Autodesk Fusion 360 part; units mm, degrees
(part 2 of 2)
sketch "Sketch7" plane through (0, 0, 4) normal (0, 0, 1) x (-1, 0, 0)
  line L0 (44.4952, -43.9167) -> (47.9684, -47.5134)
  arc A0 (45.8104, -49.5974) -> (47.9684, -47.5134) centre (46.8894, -48.5554) ccw
  line L1 (45.8104, -49.5974) -> (42.3371, -46.0007)
  arc A1 (44.4952, -43.9167) -> (42.3371, -46.0007) centre (43.4161, -44.9587) ccw
  line L2 (54.8766, -29.951) -> (59.2067, -32.451)
  arc A2 (57.7067, -35.049) -> (59.2067, -32.451) centre (58.4567, -33.75) ccw
  line L3 (57.7067, -35.049) -> (53.3766, -32.549)
  arc A3 (54.8766, -29.951) -> (53.3766, -32.549) centre (54.1266, -31.25) ccw
  line L4 (56.8322, -26.05) -> (61.3262, -28.2419)
  arc A4 (60.011, -30.9382) -> (61.3262, -28.2419) centre (60.6686, -29.5901) ccw
  line L5 (60.011, -30.9382) -> (55.5171, -28.7464)
  arc A5 (56.8322, -26.05) -> (55.5171, -28.7464) centre (56.1746, -27.3982) ccw
  line L6 (61.811, -9.3758) -> (66.735, -10.244)
  arc A6 (66.2141, -13.1985) -> (66.735, -10.244) centre (66.4745, -11.7213) ccw
  line L7 (66.2141, -13.1985) -> (61.29, -12.3302)
  arc A7 (61.811, -9.3758) -> (61.29, -12.3302) centre (61.5505, -10.853) ccw
  line L8 (58.9775, 20.7401) -> (63.7328, 22.2852)
  arc A8 (64.6598, 19.4321) -> (63.7328, 22.2852) centre (64.1963, 20.8586) ccw
  line L9 (64.6598, 19.4321) -> (59.9046, 17.887)
  arc A9 (58.9775, 20.7401) -> (59.9046, 17.887) centre (59.441, 19.3136) ccw
  circle A10 centre (0, 0) radius 15
  line L10 (60.2806, 16.5756) -> (65.1321, 17.7852)
  arc A11 (65.8578, 14.8743) -> (65.1321, 17.7852) centre (65.495, 16.3297) ccw
  line L11 (65.8578, 14.8743) -> (61.0064, 13.6647)
  arc A12 (60.2806, 16.5756) -> (61.0064, 13.6647) centre (60.6435, 15.1201) ccw
  line L12 (62.0008, 8.0248) -> (66.9734, 8.5475)
  arc A13 (67.287, 5.5639) -> (66.9734, 8.5475) centre (67.1302, 7.0557) ccw
  line L13 (67.287, 5.5639) -> (62.3144, 5.0412)
  arc A14 (62.0008, 8.0248) -> (62.3144, 5.0412) centre (62.1576, 6.533) ccw
  line L14 (61.0064, -13.6647) -> (65.8578, -14.8743)
  arc A15 (65.1321, -17.7852) -> (65.8578, -14.8743) centre (65.495, -16.3297) ccw
  line L15 (65.1321, -17.7852) -> (60.2806, -16.5756)
  arc A16 (61.0064, -13.6647) -> (60.2806, -16.5756) centre (60.6435, -15.1201) ccw
  line L16 (58.5109, -22.0221) -> (63.1468, -23.8952)
  arc A17 (62.023, -26.6767) -> (63.1468, -23.8952) centre (62.5849, -25.2859) ccw
  line L17 (62.023, -26.6767) -> (57.3871, -24.8037)
  arc A18 (58.5109, -22.0221) -> (57.3871, -24.8037) centre (57.949, -23.4129) ccw
  line L18 (57.3871, 24.8037) -> (62.023, 26.6767)
  arc A19 (63.1468, 23.8952) -> (62.023, 26.6767) centre (62.5849, 25.2859) ccw
  line L19 (63.1468, 23.8952) -> (58.5109, 22.0221)
  arc A20 (57.3871, 24.8037) -> (58.5109, 22.0221) centre (57.949, 23.4129) ccw
  line L20 (52.6536, -33.706) -> (56.7988, -36.502)
  arc A21 (55.1212, -38.9891) -> (56.7988, -36.502) centre (55.96, -37.7455) ccw
  line L21 (55.1212, -38.9891) -> (50.9761, -36.1931)
  arc A22 (52.6536, -33.706) -> (50.9761, -36.1931) centre (51.8148, -34.9496) ccw
  line L22 (47.4502, -40.7059) -> (51.166, -44.0516)
  arc A23 (49.1586, -46.281) -> (51.166, -44.0516) centre (50.1623, -45.1663) ccw
  line L23 (49.1586, -46.281) -> (45.4429, -42.9354)
  arc A24 (47.4502, -40.7059) -> (45.4429, -42.9354) centre (46.4466, -41.8207) ccw
  line L24 (62.4096, 3.6803) -> (67.4065, 3.8548)
  arc A25 (67.5112, 0.8566) -> (67.4065, 3.8548) centre (67.4589, 2.3557) ccw
  line L25 (67.5112, 0.8566) -> (62.5143, 0.6821)
  arc A26 (62.4096, 3.6803) -> (62.5143, 0.6821) centre (62.4619, 2.1812) ccw
  line L26 (62.5143, -0.6821) -> (67.5112, -0.8566)
  arc A27 (67.4065, -3.8548) -> (67.5112, -0.8566) centre (67.4589, -2.3557) ccw
  line L27 (67.4065, -3.8548) -> (62.4096, -3.6803)
  arc A28 (62.5143, -0.6821) -> (62.4096, -3.6803) centre (62.4619, -2.1812) ccw
  line L28 (62.3144, -5.0412) -> (67.287, -5.5639)
  arc A29 (66.9734, -8.5475) -> (67.287, -5.5639) centre (67.1302, -7.0557) ccw
  line L29 (66.9734, -8.5475) -> (62.0008, -8.0248)
  arc A30 (62.3144, -5.0412) -> (62.0008, -8.0248) centre (62.1576, -6.533) ccw
  line L30 (55.5171, 28.7464) -> (60.011, 30.9382)
  arc A31 (61.3262, 28.2419) -> (60.011, 30.9382) centre (60.6686, 29.5901) ccw
  line L31 (61.3262, 28.2419) -> (56.8322, 26.05)
  arc A32 (55.5171, 28.7464) -> (56.8322, 26.05) centre (56.1746, 27.3982) ccw
  line L32 (61.29, 12.3302) -> (66.2141, 13.1985)
  arc A33 (66.735, 10.244) -> (66.2141, 13.1985) centre (66.4745, 11.7213) ccw
  line L33 (66.735, 10.244) -> (61.811, 9.3758)
  arc A34 (61.29, 12.3302) -> (61.811, 9.3758) centre (61.5505, 10.853) ccw
  line L34 (59.9046, -17.887) -> (64.6598, -19.4321)
  arc A35 (63.7328, -22.2852) -> (64.6598, -19.4321) centre (64.1963, -20.8586) ccw
  line L35 (63.7328, -22.2852) -> (58.9775, -20.7401)
  arc A36 (59.9046, -17.887) -> (58.9775, -20.7401) centre (59.441, -19.3136) ccw
  circle A37 centre (47.4149, 27.375) radius 2.45
  circle A38 centre (0, -54.75) radius 2.45
  line L36 (53.3766, 32.549) -> (57.7067, 35.049)
  arc A39 (59.2067, 32.451) -> (57.7067, 35.049) centre (58.4567, 33.75) ccw
  line L37 (59.2067, 32.451) -> (54.8766, 29.951)
  arc A40 (53.3766, 32.549) -> (54.8766, 29.951) centre (54.1266, 31.25) ccw
  circle A41 centre (-47.4149, 27.375) radius 2.45
  line L38 (50.9761, 36.1931) -> (55.1212, 38.9891)
  arc A42 (56.7988, 36.502) -> (55.1212, 38.9891) centre (55.96, 37.7455) ccw
  line L39 (56.7988, 36.502) -> (52.6536, 33.706)
  arc A43 (50.9761, 36.1931) -> (52.6536, 33.706) centre (51.8148, 34.9496) ccw
  line L40 (48.3272, 39.6609) -> (52.2672, 42.7392)
  arc A44 (54.1142, 40.3751) -> (52.2672, 42.7392) centre (53.1907, 41.5571) ccw
  line L41 (54.1142, 40.3751) -> (50.1742, 37.2968)
  arc A45 (48.3272, 39.6609) -> (50.1742, 37.2968) centre (49.2507, 38.4788) ccw
  line L42 (24.5122, 4.9145) -> (55.4976, 22.8039)
  arc A46 (8, -59.4643) -> (55.4976, 22.8039) centre (0, 0) ccw
  line L43 (8, -59.4643) -> (8, -23.6854)
  arc A47 (8, -23.6854) -> (24.5122, 4.9145) centre (0, 0) ccw
  line L44 (50.1742, -37.2968) -> (54.1142, -40.3751)
  arc A48 (52.2672, -42.7392) -> (54.1142, -40.3751) centre (53.1907, -41.5571) ccw
  line L45 (52.2672, -42.7392) -> (48.3272, -39.6609)
  arc A49 (50.1742, -37.2968) -> (48.3272, -39.6609) centre (49.2507, -38.4788) ccw
  arc A50 (-7.9088, 67.0519) -> (-10.8796, 66.6343) centre (-9.3942, 66.8431) ccw
  line L46 (-7.9088, 67.0519) -> (-7.2129, 62.1005)
  arc A51 (-10.1837, 61.683) -> (-7.2129, 62.1005) centre (-8.6983, 61.8918) ccw
  line L47 (-10.1837, 61.683) -> (-10.8796, 66.6343)
  arc A52 (-3.2122, 67.4402) -> (-6.2049, 67.2309) centre (-4.7086, 67.3356) ccw
  line L48 (-3.2122, 67.4402) -> (-2.8634, 62.4524)
  arc A53 (-5.8561, 62.2431) -> (-2.8634, 62.4524) centre (-4.3598, 62.3478) ccw
  line L49 (-5.8561, 62.2431) -> (-6.2049, 67.2309)
  line L50 (-1.5, 62.5) -> (-1.5, 67.5)
  arc A54 (1.5, 67.5) -> (-1.5, 67.5) centre (0, 67.5) ccw
  line L51 (1.5, 67.5) -> (1.5, 62.5)
  arc A55 (-1.5, 62.5) -> (1.5, 62.5) centre (0, 62.5) ccw
  line L52 (2.8634, 62.4524) -> (3.2122, 67.4402)
  arc A56 (6.2049, 67.2309) -> (3.2122, 67.4402) centre (4.7086, 67.3356) ccw
  line L53 (6.2049, 67.2309) -> (5.8561, 62.2431)
  arc A57 (2.8634, 62.4524) -> (5.8561, 62.2431) centre (4.3598, 62.3478) ccw
  line L54 (7.2129, 62.1005) -> (7.9088, 67.0519)
  arc A58 (10.8796, 66.6343) -> (7.9088, 67.0519) centre (9.3942, 66.8431) ccw
  line L55 (10.8796, 66.6343) -> (10.1837, 61.683)
  arc A59 (7.2129, 62.1005) -> (10.1837, 61.683) centre (8.6983, 61.8918) ccw
  line L56 (11.5273, 61.4461) -> (12.5668, 66.3368)
  arc A60 (15.5013, 65.7131) -> (12.5668, 66.3368) centre (14.034, 66.025) ccw
  line L57 (15.5013, 65.7131) -> (14.4617, 60.8224)
  arc A61 (11.5273, 61.4461) -> (14.4617, 60.8224) centre (12.9945, 61.1342) ccw
  line L58 (15.7854, 60.4923) -> (17.1636, 65.2986)
  arc A62 (20.0474, 64.4717) -> (17.1636, 65.2986) centre (18.6055, 64.8852) ccw
  line L59 (20.0474, 64.4717) -> (18.6692, 59.6654)
  arc A63 (15.7854, 60.4923) -> (18.6692, 59.6654) centre (17.2273, 60.0789) ccw
  line L60 (19.9667, 59.2438) -> (21.6768, 63.9423)
  arc A64 (24.4959, 62.9162) -> (21.6768, 63.9423) centre (23.0864, 63.4293) ccw
  line L61 (24.4959, 62.9162) -> (22.7858, 58.2178)
  arc A65 (19.9667, 59.2438) -> (22.7858, 58.2178) centre (21.3763, 58.7308) ccw
  line L62 (24.0507, 57.7067) -> (26.0844, 62.2744)
  arc A66 (28.825, 61.0542) -> (26.0844, 62.2744) centre (27.4547, 61.6643) ccw
  line L63 (28.825, 61.0542) -> (26.7914, 56.4865)
  arc A67 (24.0507, 57.7067) -> (26.7914, 56.4865) centre (25.421, 57.0966) ccw
  line L64 (28.0176, 55.8884) -> (30.3649, 60.3032)
  arc A68 (33.0138, 58.8948) -> (30.3649, 60.3032) centre (31.6893, 59.599) ccw
  line L65 (33.0138, 58.8948) -> (30.6664, 54.48)
  arc A69 (28.0176, 55.8884) -> (30.6664, 54.48) centre (29.342, 55.1842) ccw
  line L66 (39.0252, 48.842) -> (42.2391, 52.6722)
  arc A70 (44.5372, 50.7438) -> (42.2391, 52.6722) centre (43.3882, 51.708) ccw
  line L67 (44.5372, 50.7438) -> (41.3233, 46.9136)
  arc A71 (39.0252, 48.842) -> (41.3233, 46.9136) centre (40.1742, 47.8778) ccw
  line L68 (31.8479, 53.7979) -> (34.4975, 58.0381)
  arc A72 (37.0416, 56.4484) -> (34.4975, 58.0381) centre (35.7696, 57.2432) ccw
  line L69 (37.0416, 56.4484) -> (34.392, 52.2081)
  arc A73 (31.8479, 53.7979) -> (34.392, 52.2081) centre (33.12, 53.003) ccw
  line L70 (45.4429, 42.9354) -> (49.1586, 46.281)
  arc A74 (51.166, 44.0516) -> (49.1586, 46.281) centre (50.1623, 45.1663) ccw
  line L71 (51.166, 44.0516) -> (47.4502, 40.7059)
  arc A75 (45.4429, 42.9354) -> (47.4502, 40.7059) centre (46.4466, 41.8207) ccw
  line L72 (42.3371, 46.0007) -> (45.8104, 49.5974)
  arc A76 (47.9684, 47.5134) -> (45.8104, 49.5974) centre (46.8894, 48.5554) ccw
  line L73 (47.9684, 47.5134) -> (44.4952, 43.9167)
  arc A77 (42.3371, 46.0007) -> (44.4952, 43.9167) centre (43.4161, 44.9587) ccw
  line L74 (35.5231, 51.4452) -> (38.462, 55.4903)
  arc A78 (40.889, 53.727) -> (38.462, 55.4903) centre (39.6755, 54.6086) ccw
  line L75 (40.889, 53.727) -> (37.9501, 49.6819)
  arc A79 (35.5231, 51.4452) -> (37.9501, 49.6819) centre (36.7366, 50.5636) ccw
  line L76 (10.1837, -61.683) -> (10.8796, -66.6343)
  arc A80 (7.9088, -67.0519) -> (10.8796, -66.6343) centre (9.3942, -66.8431) ccw
  line L77 (7.9088, -67.0519) -> (7.2129, -62.1005)
  arc A81 (10.1837, -61.683) -> (7.2129, -62.1005) centre (8.6983, -61.8918) ccw
  line L78 (14.4617, -60.8224) -> (15.5013, -65.7131)
  arc A82 (12.5668, -66.3368) -> (15.5013, -65.7131) centre (14.034, -66.025) ccw
  line L79 (12.5668, -66.3368) -> (11.5273, -61.4461)
  arc A83 (14.4617, -60.8224) -> (11.5273, -61.4461) centre (12.9945, -61.1342) ccw
  line L80 (5.8561, -62.2431) -> (6.2049, -67.2309)
  arc A84 (3.2122, -67.4402) -> (6.2049, -67.2309) centre (4.7086, -67.3356) ccw
  line L81 (3.2122, -67.4402) -> (2.8634, -62.4524)
  arc A85 (5.8561, -62.2431) -> (2.8634, -62.4524) centre (4.3598, -62.3478) ccw
  line L82 (18.6692, -59.6654) -> (20.0474, -64.4717)
  arc A86 (17.1636, -65.2986) -> (20.0474, -64.4717) centre (18.6055, -64.8852) ccw
  line L83 (17.1636, -65.2986) -> (15.7854, -60.4923)
  arc A87 (18.6692, -59.6654) -> (15.7854, -60.4923) centre (17.2273, -60.0789) ccw
  line L84 (22.7858, -58.2178) -> (24.4959, -62.9162)
  arc A88 (21.6768, -63.9423) -> (24.4959, -62.9162) centre (23.0864, -63.4293) ccw
  line L85 (21.6768, -63.9423) -> (19.9667, -59.2438)
  arc A89 (22.7858, -58.2178) -> (19.9667, -59.2438) centre (21.3763, -58.7308) ccw
  line L86 (26.7914, -56.4865) -> (28.825, -61.0542)
  arc A90 (26.0844, -62.2744) -> (28.825, -61.0542) centre (27.4547, -61.6643) ccw
  line L87 (26.0844, -62.2744) -> (24.0507, -57.7067)
  arc A91 (26.7914, -56.4865) -> (24.0507, -57.7067) centre (25.421, -57.0966) ccw
  line L88 (30.6664, -54.48) -> (33.0138, -58.8948)
  arc A92 (30.3649, -60.3032) -> (33.0138, -58.8948) centre (31.6893, -59.599) ccw
  line L89 (30.3649, -60.3032) -> (28.0176, -55.8884)
  arc A93 (30.6664, -54.48) -> (28.0176, -55.8884) centre (29.342, -55.1842) ccw
  line L90 (34.392, -52.2081) -> (37.0416, -56.4484)
  arc A94 (34.4975, -58.0381) -> (37.0416, -56.4484) centre (35.7696, -57.2432) ccw
  line L91 (34.4975, -58.0381) -> (31.8479, -53.7979)
  arc A95 (34.392, -52.2081) -> (31.8479, -53.7979) centre (33.12, -53.003) ccw
  line L92 (37.9501, -49.6819) -> (40.889, -53.727)
  arc A96 (38.462, -55.4903) -> (40.889, -53.727) centre (39.6755, -54.6086) ccw
  line L93 (38.462, -55.4903) -> (35.5231, -51.4452)
  arc A97 (37.9501, -49.6819) -> (35.5231, -51.4452) centre (36.7366, -50.5636) ccw
  line L94 (41.3233, -46.9136) -> (44.5372, -50.7438)
  arc A98 (42.2391, -52.6722) -> (44.5372, -50.7438) centre (43.3882, -51.708) ccw
  line L95 (42.2391, -52.6722) -> (39.0252, -48.842)
  arc A99 (41.3233, -46.9136) -> (39.0252, -48.842) centre (40.1742, -47.8778) ccw
  line L96 (1.5, -62.5) -> (1.5, -67.5)
  arc A100 (-1.5, -67.5) -> (1.5, -67.5) centre (0, -67.5) ccw
  line L97 (-1.5, -67.5) -> (-1.5, -62.5)
  arc A101 (1.5, -62.5) -> (-1.5, -62.5) centre (0, -62.5) ccw
  arc A102 (-6.2049, -67.2309) -> (-3.2122, -67.4402) centre (-4.7086, -67.3356) ccw
  line L98 (-6.2049, -67.2309) -> (-5.8561, -62.2431)
  arc A103 (-2.8634, -62.4524) -> (-5.8561, -62.2431) centre (-4.3598, -62.3478) ccw
  line L99 (-2.8634, -62.4524) -> (-3.2122, -67.4402)
  arc A104 (-55.4976, 22.8039) -> (-8, -59.4643) centre (0, 0) ccw
  line L100 (-55.4976, 22.8039) -> (-24.5122, 4.9145)
  arc A105 (-24.5122, 4.9145) -> (-8, -23.6854) centre (0, 0) ccw
  line L101 (-8, -23.6854) -> (-8, -59.4643)
  arc A106 (-10.8796, -66.6343) -> (-7.9088, -67.0519) centre (-9.3942, -66.8431) ccw
  line L102 (-10.8796, -66.6343) -> (-10.1837, -61.683)
  arc A107 (-7.2129, -62.1005) -> (-10.1837, -61.683) centre (-8.6983, -61.8918) ccw
  line L103 (-7.2129, -62.1005) -> (-7.9088, -67.0519)
  arc A108 (-15.5013, -65.7131) -> (-12.5668, -66.3368) centre (-14.034, -66.025) ccw
  line L104 (-15.5013, -65.7131) -> (-14.4617, -60.8224)
  arc A109 (-11.5273, -61.4461) -> (-14.4617, -60.8224) centre (-12.9945, -61.1342) ccw
  line L105 (-11.5273, -61.4461) -> (-12.5668, -66.3368)
  arc A110 (-20.0474, -64.4717) -> (-17.1636, -65.2986) centre (-18.6055, -64.8852) ccw
  line L106 (-20.0474, -64.4717) -> (-18.6692, -59.6654)
  arc A111 (-15.7854, -60.4923) -> (-18.6692, -59.6654) centre (-17.2273, -60.0789) ccw
  line L107 (-15.7854, -60.4923) -> (-17.1636, -65.2986)
  arc A112 (-24.4959, -62.9162) -> (-21.6768, -63.9423) centre (-23.0864, -63.4293) ccw
  line L108 (-24.4959, -62.9162) -> (-22.7858, -58.2178)
  arc A113 (-19.9667, -59.2438) -> (-22.7858, -58.2178) centre (-21.3763, -58.7308) ccw
  line L109 (-19.9667, -59.2438) -> (-21.6768, -63.9423)
  arc A114 (-28.825, -61.0542) -> (-26.0844, -62.2744) centre (-27.4547, -61.6643) ccw
  line L110 (-28.825, -61.0542) -> (-26.7914, -56.4865)
  arc A115 (-24.0507, -57.7067) -> (-26.7914, -56.4865) centre (-25.421, -57.0966) ccw
  line L111 (-24.0507, -57.7067) -> (-26.0844, -62.2744)
  arc A116 (-33.0138, -58.8948) -> (-30.3649, -60.3032) centre (-31.6893, -59.599) ccw
  line L112 (-33.0138, -58.8948) -> (-30.6664, -54.48)
  arc A117 (-28.0176, -55.8884) -> (-30.6664, -54.48) centre (-29.342, -55.1842) ccw
  line L113 (-28.0176, -55.8884) -> (-30.3649, -60.3032)
  arc A118 (-37.0416, -56.4484) -> (-34.4975, -58.0381) centre (-35.7696, -57.2432) ccw
  line L114 (-37.0416, -56.4484) -> (-34.392, -52.2081)
  arc A119 (-31.8479, -53.7979) -> (-34.392, -52.2081) centre (-33.12, -53.003) ccw
  line L115 (-31.8479, -53.7979) -> (-34.4975, -58.0381)
  arc A120 (-40.889, -53.727) -> (-38.462, -55.4903) centre (-39.6755, -54.6086) ccw
  line L116 (-40.889, -53.727) -> (-37.9501, -49.6819)
  arc A121 (-35.5231, -51.4452) -> (-37.9501, -49.6819) centre (-36.7366, -50.5636) ccw
  line L117 (-35.5231, -51.4452) -> (-38.462, -55.4903)
  arc A122 (-44.5372, -50.7438) -> (-42.2391, -52.6722) centre (-43.3882, -51.708) ccw
  line L118 (-44.5372, -50.7438) -> (-41.3233, -46.9136)
  arc A123 (-39.0252, -48.842) -> (-41.3233, -46.9136) centre (-40.1742, -47.8778) ccw
  line L119 (-39.0252, -48.842) -> (-42.2391, -52.6722)
  arc A124 (-47.9684, -47.5134) -> (-45.8104, -49.5974) centre (-46.8894, -48.5554) ccw
  line L120 (-47.9684, -47.5134) -> (-44.4952, -43.9167)
  arc A125 (-42.3371, -46.0007) -> (-44.4952, -43.9167) centre (-43.4161, -44.9587) ccw
  line L121 (-42.3371, -46.0007) -> (-45.8104, -49.5974)
  arc A126 (-51.166, -44.0516) -> (-49.1586, -46.281) centre (-50.1623, -45.1663) ccw
  line L122 (-51.166, -44.0516) -> (-47.4502, -40.7059)
  arc A127 (-45.4429, -42.9354) -> (-47.4502, -40.7059) centre (-46.4466, -41.8207) ccw
  line L123 (-45.4429, -42.9354) -> (-49.1586, -46.281)
  arc A128 (-54.1142, -40.3751) -> (-52.2672, -42.7392) centre (-53.1907, -41.5571) ccw
  line L124 (-54.1142, -40.3751) -> (-50.1742, -37.2968)
  arc A129 (-48.3272, -39.6609) -> (-50.1742, -37.2968) centre (-49.2507, -38.4788) ccw
  line L125 (-48.3272, -39.6609) -> (-52.2672, -42.7392)
  arc A130 (-56.7988, -36.502) -> (-55.1212, -38.9891) centre (-55.96, -37.7455) ccw
  line L126 (-56.7988, -36.502) -> (-52.6536, -33.706)
  arc A131 (-50.9761, -36.1931) -> (-52.6536, -33.706) centre (-51.8148, -34.9496) ccw
  line L127 (-50.9761, -36.1931) -> (-55.1212, -38.9891)
  arc A132 (-59.2067, -32.451) -> (-57.7067, -35.049) centre (-58.4567, -33.75) ccw
  line L128 (-59.2067, -32.451) -> (-54.8766, -29.951)
  arc A133 (-53.3766, -32.549) -> (-54.8766, -29.951) centre (-54.1266, -31.25) ccw
  line L129 (-53.3766, -32.549) -> (-57.7067, -35.049)
  arc A134 (-61.3262, -28.2419) -> (-60.011, -30.9382) centre (-60.6686, -29.5901) ccw
  line L130 (-61.3262, -28.2419) -> (-56.8322, -26.05)
  arc A135 (-55.5171, -28.7464) -> (-56.8322, -26.05) centre (-56.1746, -27.3982) ccw
  line L131 (-55.5171, -28.7464) -> (-60.011, -30.9382)
  arc A136 (-63.1468, -23.8952) -> (-62.023, -26.6767) centre (-62.5849, -25.2859) ccw
  line L132 (-63.1468, -23.8952) -> (-58.5109, -22.0221)
  arc A137 (-57.3871, -24.8037) -> (-58.5109, -22.0221) centre (-57.949, -23.4129) ccw
  line L133 (-57.3871, -24.8037) -> (-62.023, -26.6767)
  arc A138 (-64.6598, -19.4321) -> (-63.7328, -22.2852) centre (-64.1963, -20.8586) ccw
  line L134 (-64.6598, -19.4321) -> (-59.9046, -17.887)
  arc A139 (-58.9775, -20.7401) -> (-59.9046, -17.887) centre (-59.441, -19.3136) ccw
  line L135 (-58.9775, -20.7401) -> (-63.7328, -22.2852)
  arc A140 (-65.8578, -14.8743) -> (-65.1321, -17.7852) centre (-65.495, -16.3297) ccw
  line L136 (-65.8578, -14.8743) -> (-61.0064, -13.6647)
  arc A141 (-60.2806, -16.5756) -> (-61.0064, -13.6647) centre (-60.6435, -15.1201) ccw
  line L137 (-60.2806, -16.5756) -> (-65.1321, -17.7852)
  arc A142 (-66.735, -10.244) -> (-66.2141, -13.1985) centre (-66.4745, -11.7213) ccw
  line L138 (-66.735, -10.244) -> (-61.811, -9.3758)
  arc A143 (-61.29, -12.3302) -> (-61.811, -9.3758) centre (-61.5505, -10.853) ccw
  line L139 (-61.29, -12.3302) -> (-66.2141, -13.1985)
  arc A144 (-67.287, -5.5639) -> (-66.9734, -8.5475) centre (-67.1302, -7.0557) ccw
  line L140 (-67.287, -5.5639) -> (-62.3144, -5.0412)
  arc A145 (-62.0008, -8.0248) -> (-62.3144, -5.0412) centre (-62.1576, -6.533) ccw
  line L141 (-62.0008, -8.0248) -> (-66.9734, -8.5475)
  arc A146 (-67.5112, -0.8566) -> (-67.4065, -3.8548) centre (-67.4589, -2.3557) ccw
  line L142 (-67.5112, -0.8566) -> (-62.5143, -0.6821)
  arc A147 (-62.4096, -3.6803) -> (-62.5143, -0.6821) centre (-62.4619, -2.1812) ccw
  line L143 (-62.4096, -3.6803) -> (-67.4065, -3.8548)
  arc A148 (-67.4065, 3.8548) -> (-67.5112, 0.8566) centre (-67.4589, 2.3557) ccw
  line L144 (-67.4065, 3.8548) -> (-62.4096, 3.6803)
  arc A149 (-62.5143, 0.6821) -> (-62.4096, 3.6803) centre (-62.4619, 2.1812) ccw
  line L145 (-62.5143, 0.6821) -> (-67.5112, 0.8566)
  arc A150 (-66.9734, 8.5475) -> (-67.287, 5.5639) centre (-67.1302, 7.0557) ccw
  line L146 (-66.9734, 8.5475) -> (-62.0008, 8.0248)
  arc A151 (-62.3144, 5.0412) -> (-62.0008, 8.0248) centre (-62.1576, 6.533) ccw
  line L147 (-62.3144, 5.0412) -> (-67.287, 5.5639)
  arc A152 (-66.2141, 13.1985) -> (-66.735, 10.244) centre (-66.4745, 11.7213) ccw
  line L148 (-66.2141, 13.1985) -> (-61.29, 12.3302)
  arc A153 (-61.811, 9.3758) -> (-61.29, 12.3302) centre (-61.5505, 10.853) ccw
  line L149 (-61.811, 9.3758) -> (-66.735, 10.244)
  arc A154 (-65.1321, 17.7852) -> (-65.8578, 14.8743) centre (-65.495, 16.3297) ccw
  line L150 (-65.1321, 17.7852) -> (-60.2806, 16.5756)
  arc A155 (-61.0064, 13.6647) -> (-60.2806, 16.5756) centre (-60.6435, 15.1201) ccw
  line L151 (-61.0064, 13.6647) -> (-65.8578, 14.8743)
  arc A156 (-63.7328, 22.2852) -> (-64.6598, 19.4321) centre (-64.1963, 20.8586) ccw
  line L152 (-63.7328, 22.2852) -> (-58.9775, 20.7401)
  arc A157 (-59.9046, 17.887) -> (-58.9775, 20.7401) centre (-59.441, 19.3136) ccw
  line L153 (-59.9046, 17.887) -> (-64.6598, 19.4321)
  arc A158 (-62.023, 26.6767) -> (-63.1468, 23.8952) centre (-62.5849, 25.2859) ccw
  line L154 (-62.023, 26.6767) -> (-57.3871, 24.8037)
  arc A159 (-58.5109, 22.0221) -> (-57.3871, 24.8037) centre (-57.949, 23.4129) ccw
  line L155 (-58.5109, 22.0221) -> (-63.1468, 23.8952)
  arc A160 (-60.011, 30.9382) -> (-61.3262, 28.2419) centre (-60.6686, 29.5901) ccw
  line L156 (-60.011, 30.9382) -> (-55.5171, 28.7464)
  arc A161 (-56.8322, 26.05) -> (-55.5171, 28.7464) centre (-56.1746, 27.3982) ccw
  line L157 (-56.8322, 26.05) -> (-61.3262, 28.2419)
  arc A162 (-57.7067, 35.049) -> (-59.2067, 32.451) centre (-58.4567, 33.75) ccw
  line L158 (-57.7067, 35.049) -> (-53.3766, 32.549)
  arc A163 (-54.8766, 29.951) -> (-53.3766, 32.549) centre (-54.1266, 31.25) ccw
  line L159 (-54.8766, 29.951) -> (-59.2067, 32.451)
  arc A164 (-55.1212, 38.9891) -> (-56.7988, 36.502) centre (-55.96, 37.7455) ccw
  line L160 (-55.1212, 38.9891) -> (-50.9761, 36.1931)
  arc A165 (-52.6536, 33.706) -> (-50.9761, 36.1931) centre (-51.8148, 34.9496) ccw
  line L161 (-52.6536, 33.706) -> (-56.7988, 36.502)
  line L162 (-16.5122, 18.7709) -> (-47.4976, 36.6603)
  arc A166 (47.4976, 36.6603) -> (-47.4976, 36.6603) centre (0, 0) ccw
  line L163 (47.4976, 36.6603) -> (16.5122, 18.7709)
  arc A167 (16.5122, 18.7709) -> (-16.5122, 18.7709) centre (0, 0) ccw
  arc A168 (-52.2672, 42.7392) -> (-54.1142, 40.3751) centre (-53.1907, 41.5571) ccw
  line L164 (-52.2672, 42.7392) -> (-48.3272, 39.6609)
  arc A169 (-50.1742, 37.2968) -> (-48.3272, 39.6609) centre (-49.2507, 38.4788) ccw
  line L165 (-50.1742, 37.2968) -> (-54.1142, 40.3751)
  arc A170 (-49.1586, 46.281) -> (-51.166, 44.0516) centre (-50.1623, 45.1663) ccw
  line L166 (-49.1586, 46.281) -> (-45.4429, 42.9354)
  arc A171 (-47.4502, 40.7059) -> (-45.4429, 42.9354) centre (-46.4466, 41.8207) ccw
  line L167 (-47.4502, 40.7059) -> (-51.166, 44.0516)
  arc A172 (-45.8104, 49.5974) -> (-47.9684, 47.5134) centre (-46.8894, 48.5554) ccw
  line L168 (-45.8104, 49.5974) -> (-42.3371, 46.0007)
  arc A173 (-44.4952, 43.9167) -> (-42.3371, 46.0007) centre (-43.4161, 44.9587) ccw
  line L169 (-44.4952, 43.9167) -> (-47.9684, 47.5134)
  arc A174 (-42.2391, 52.6722) -> (-44.5372, 50.7438) centre (-43.3882, 51.708) ccw
  line L170 (-42.2391, 52.6722) -> (-39.0252, 48.842)
  arc A175 (-41.3233, 46.9136) -> (-39.0252, 48.842) centre (-40.1742, 47.8778) ccw
  line L171 (-41.3233, 46.9136) -> (-44.5372, 50.7438)
  arc A176 (-38.462, 55.4903) -> (-40.889, 53.727) centre (-39.6755, 54.6086) ccw
  line L172 (-38.462, 55.4903) -> (-35.5231, 51.4452)
  arc A177 (-37.9501, 49.6819) -> (-35.5231, 51.4452) centre (-36.7366, 50.5636) ccw
  line L173 (-37.9501, 49.6819) -> (-40.889, 53.727)
  arc A178 (-34.4975, 58.0381) -> (-37.0416, 56.4484) centre (-35.7696, 57.2432) ccw
  line L174 (-34.4975, 58.0381) -> (-31.8479, 53.7979)
  arc A179 (-34.392, 52.2081) -> (-31.8479, 53.7979) centre (-33.12, 53.003) ccw
  line L175 (-34.392, 52.2081) -> (-37.0416, 56.4484)
  arc A180 (-30.3649, 60.3032) -> (-33.0138, 58.8948) centre (-31.6893, 59.599) ccw
  line L176 (-30.3649, 60.3032) -> (-28.0176, 55.8884)
  arc A181 (-30.6664, 54.48) -> (-28.0176, 55.8884) centre (-29.342, 55.1842) ccw
  line L177 (-30.6664, 54.48) -> (-33.0138, 58.8948)
  arc A182 (-26.0844, 62.2744) -> (-28.825, 61.0542) centre (-27.4547, 61.6643) ccw
  line L178 (-26.0844, 62.2744) -> (-24.0507, 57.7067)
  arc A183 (-26.7914, 56.4865) -> (-24.0507, 57.7067) centre (-25.421, 57.0966) ccw
  line L179 (-26.7914, 56.4865) -> (-28.825, 61.0542)
  arc A184 (-21.6768, 63.9423) -> (-24.4959, 62.9162) centre (-23.0864, 63.4293) ccw
  line L180 (-21.6768, 63.9423) -> (-19.9667, 59.2438)
  arc A185 (-22.7858, 58.2178) -> (-19.9667, 59.2438) centre (-21.3763, 58.7308) ccw
  line L181 (-22.7858, 58.2178) -> (-24.4959, 62.9162)
  arc A186 (-17.1636, 65.2986) -> (-20.0474, 64.4717) centre (-18.6055, 64.8852) ccw
  line L182 (-17.1636, 65.2986) -> (-15.7854, 60.4923)
  arc A187 (-18.6692, 59.6654) -> (-15.7854, 60.4923) centre (-17.2273, 60.0789) ccw
  line L183 (-18.6692, 59.6654) -> (-20.0474, 64.4717)
  arc A188 (-12.5668, 66.3368) -> (-15.5013, 65.7131) centre (-14.034, 66.025) ccw
  line L184 (-12.5668, 66.3368) -> (-11.5273, 61.4461)
  arc A189 (-14.4617, 60.8224) -> (-11.5273, 61.4461) centre (-12.9945, 61.1342) ccw
  line L185 (-14.4617, 60.8224) -> (-15.5013, 65.7131)
  circle A190 centre (0, 0) radius 70
  line L186 (-2.2228, -50.9) -> (-4.4456, -54.75)
  line L187 (-4.4456, -54.75) -> (-2.2228, -58.6)
  line L188 (-2.2228, -58.6) -> (2.2228, -58.6)
  line L189 (2.2228, -58.6) -> (4.4456, -54.75)
  line L190 (4.4456, -54.75) -> (2.2228, -50.9)
  line L191 (2.2228, -50.9) -> (-2.2228, -50.9)
  line L192 (45.1921, 23.525) -> (49.6377, 23.525)
  line L193 (49.6377, 23.525) -> (51.8605, 27.375)
  line L194 (51.8605, 27.375) -> (49.6377, 31.225)
  line L195 (49.6377, 31.225) -> (45.1921, 31.225)
  line L196 (45.1921, 31.225) -> (42.9693, 27.375)
  line L197 (42.9693, 27.375) -> (45.1921, 23.525)
  circle A191 centre (47.4149, 27.375) radius 2.45
  line L198 (-42.9693, 27.375) -> (-45.1921, 31.225)
  line L199 (-45.1921, 31.225) -> (-49.6377, 31.225)
  line L200 (-49.6377, 31.225) -> (-51.8605, 27.375)
  line L201 (-51.8605, 27.375) -> (-49.6377, 23.525)
  line L202 (-49.6377, 23.525) -> (-45.1921, 23.525)
  line L203 (-45.1921, 23.525) -> (-42.9693, 27.375)
  circle A192 centre (-47.4149, 27.375) radius 2.45
  point P0 (0, -54.75)
  dimension "d48" = 7.7
  dimension "d50" = 360
  constraint coincident P0 A38.centre
  constraint horizontal L191
  measures "d48" distance of L188 L191
extrude "Extrude6" add sketch "Sketch7" along normal blind 7 contours L186 L187 L188 L189 L190 L191 | L192 L193 L194 L195 L196 L197 | L198 L199 L200 L201 L202 L203
equation "d31 = 43.4 mm + ( 14.8 / 2 ) * 1 mm"
